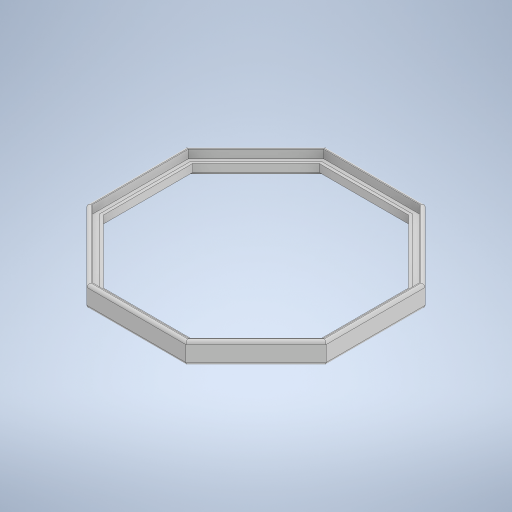
# Autodesk Inventor part: OV-PAM_ring_2
Saved by Autodesk Inventor 2024 (Build 280153000, 153)
## iProperties
Created: 2023-06-19
Part Number: OV-PAM_ring_2
Material: 일반
Document SubType Name: Modeling
Designer: jsw
Density: 1 g/cm^3
Appearance: 기본값
Author: jsw
Autodesk Inventor part; units mm, degrees
ref_plane "YZ Plane" through (0, 0, 0) normal (1, 0, 0) x (0, 1, 0)
ref_plane "XZ Plane" through (0, 0, 0) normal (0, 1, 0) x (-1, 0, 0)
ref_plane "XY Plane" through (0, 0, 0) normal (0, 0, 1) x (1, 0, 0)
sketch "스케치1" plane through (0, 0, 0) normal (0, 1, 0) x (-1, 0, 0)
  line L0 (-46.0919, 19.0919) -> (-19.0919, 46.0919)
  line L1 (-19.0919, 46.0919) -> (19.0919, 46.0919)
  line L2 (19.0919, 46.0919) -> (46.0919, 19.0919)
  line L3 (46.0919, 19.0919) -> (46.0919, -19.0919)
  line L4 (46.0919, -19.0919) -> (19.0919, -46.0919)
  line L5 (19.0919, -46.0919) -> (-19.0919, -46.0919)
  line L6 (-19.0919, -46.0919) -> (-46.0919, -19.0919)
  line L7 (-46.0919, -19.0919) -> (-46.0919, 19.0919)
  line L8 (49.2919, 20.4174) -> (49.2919, -20.4174)
  line L9 (49.2919, -20.4174) -> (20.4174, -49.2919)
  line L10 (20.4174, -49.2919) -> (-20.4174, -49.2919)
  line L11 (-20.4174, -49.2919) -> (-49.2919, -20.4174)
  line L12 (-49.2919, -20.4174) -> (-49.2919, 20.4174)
  line L13 (-49.2919, 20.4174) -> (-20.4174, 49.2919)
  line L14 (-20.4174, 49.2919) -> (20.4174, 49.2919)
  line L15 (20.4174, 49.2919) -> (49.2919, 20.4174)
  point P0 (0, 0)
  point P1 (0, 0)
  point P2 (0, 0)
  dimension "d0" = 38.1838
  dimension "d1" = 3.2
  constraints: 32 end point, 2 coincident, 2 horizontal, 34 other
  measures "d0" distance of L2.end L3.end
  measures "d1" distance between parallel lines of L8 L3
extrude "돌출1" add sketch "스케치1" along normal blind 8.8 contours L0 L1 L2 L3 L4 L5 L6 L7 | L8 L9 L10 L11 L12 L13 L14 L15
sketch "스케치3" plane through (0, 0, 0) normal (0, -1, 0) x (1, 0, 0)
  line L0 (-18.9262, 45.6919) -> (18.9262, 45.6919)
  line L1 (18.9262, 45.6919) -> (45.6919, 18.9262)
  line L2 (45.6919, 18.9262) -> (45.6919, -18.9262)
  line L3 (45.6919, -18.9262) -> (18.9262, -45.6919)
  line L4 (18.9262, -45.6919) -> (-18.9262, -45.6919)
  line L5 (-18.9262, -45.6919) -> (-45.6919, -18.9262)
  line L6 (-45.6919, -18.9262) -> (-45.6919, 18.9262)
  line L7 (-45.6919, 18.9262) -> (-18.9262, 45.6919)
  line L8 (-19.7546, 47.6919) -> (19.7546, 47.6919)
  line L9 (19.7546, 47.6919) -> (47.6919, 19.7546)
  line L10 (47.6919, 19.7546) -> (47.6919, -19.7546)
  line L11 (47.6919, -19.7546) -> (19.7546, -47.6919)
  line L12 (19.7546, -47.6919) -> (-19.7546, -47.6919)
  line L13 (-19.7546, -47.6919) -> (-47.6919, -19.7546)
  line L14 (-47.6919, -19.7546) -> (-47.6919, 19.7546)
  line L15 (-47.6919, 19.7546) -> (-19.7546, 47.6919)
  line L16 (-20.4174, 49.2919) -> (20.4174, 49.2919) projected
  point P0 (0, 0)
  point P1 (0, 0)
  point P2 (0, 0)
  point P3 (0, 0)
  dimension "d9" = 2
  dimension "d144" = 1.6
  constraints: 32 end point, 3 coincident, 2 horizontal, 34 other
  measures "d9" distance between parallel lines of L8 L0
  measures "d144" distance between parallel lines of L8 L16
extrude "돌출3" cut sketch "스케치3" against normal blind 3.4
sketch "스케치14" plane through (0, 0, 0) normal (0, -1, 0) x (1, 0, 0)
  line L0 (45.6919, 18.9262) -> (18.9262, 45.6919) projected
  line L1 (18.9262, 45.6919) -> (-18.9262, 45.6919) projected
  line L2 (-18.9262, 45.6919) -> (-45.6919, 18.9262) projected
  line L3 (-45.6919, 18.9262) -> (-45.6919, -18.9262) projected
  line L4 (-45.6919, -18.9262) -> (-18.9262, -45.6919) projected
  line L5 (-18.9262, -45.6919) -> (18.9262, -45.6919) projected
  line L6 (18.9262, -45.6919) -> (45.6919, -18.9262) projected
  line L7 (45.6919, -18.9262) -> (45.6919, 18.9262) projected
  point P0 (0, 0)
extrude "돌출16" cut sketch "스케치14" against normal blind 2.8
sketch "스케치15" plane through (0, 2.8, 0) normal (0, -1, 0) x (1, 0, 0)
  line L0 (-18.4291, 44.4919) -> (18.4291, 44.4919)
  line L1 (18.4291, 44.4919) -> (44.4919, 18.4291)
  line L2 (44.4919, 18.4291) -> (44.4919, -18.4291)
  line L3 (44.4919, -18.4291) -> (18.4291, -44.4919)
  line L4 (18.4291, -44.4919) -> (-18.4291, -44.4919)
  line L5 (-18.4291, -44.4919) -> (-44.4919, -18.4291)
  line L6 (-44.4919, -18.4291) -> (-44.4919, 18.4291)
  line L7 (-44.4919, 18.4291) -> (-18.4291, 44.4919)
  line L8 (-18.9262, 45.6919) -> (18.9262, 45.6919) projected
  point P0 (0, 0)
  point P1 (0, 0)
  dimension "d140" = 1.2
  constraints: 16 end point, 1 coincident, 1 horizontal, 17 other
  measures "d140" distance between parallel lines of L0 L8
extrude "돌출17" cut sketch "스케치15" against normal up to surface (6 mm away)
ref_plane "작업 평면3" through (0, 4.4, 0) normal (0, -1, 0) x (1, 0, 0)
mirror "미러6" about plane through (0, 4.4, 0) normal (0, -1, 0) of "돌출3", "돌출16"
fillet "모깎기2" radius 1.2 16 edges at (0, 0, 49.2919) (-34.8546, 0, 34.8546) (-49.2919, 0, 0) (-34.8546, 0, -34.8546) (0, 0, -49.2919) (34.8546, 0, -34.8546) (49.2919, 0, 0) (34.8546, 0, 34.8546) (-34.8546, 8.8, 34.8546) (-49.2919, 8.8, 0) (-34.8546, 8.8, -34.8546) (0, 8.8, -49.2919) (34.8546, 8.8, -34.8546) (49.2919, 8.8, 0) (34.8546, 8.8, 34.8546) (0, 8.8, 49.2919)
